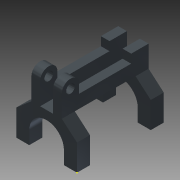
# Autodesk Inventor part: HW 4 Part 4
Saved by Autodesk Inventor 2015 (Build 190159000, 159)
## iProperties
Created: 2016-01-31
Part Number: HW 4 Part 4
Material: Iron, Cast
Document SubType Name: Modeling
Designer: Melissa
Mass: 1308.22 g
Surface Area: 443.91 cm^2
Volume: 182.968 cm^3
Density: 7.15 g/cm^3
Appearance: Iron Gray
Author: Melissa
Autodesk Inventor part; units mm, degrees
ref_plane "YZ Plane" through (0, 0, 0) normal (1, 0, 0) x (0, 1, 0)
ref_plane "XZ Plane" through (0, 0, 0) normal (0, 1, 0) x (-1, 0, 0)
ref_plane "XY Plane" through (0, 0, 0) normal (0, 0, 1) x (1, 0, 0)
sketch "Sketch1" plane through (0, 0, 0) normal (0, 0, 1) x (1, 0, 0)
  line L0 (0, 0) -> (19.05, 0)
  line L1 (19.05, 0) -> (19.05, 19.05)
  line L2 (69.85, 19.05) -> (69.85, 0)
  line L3 (69.85, 0) -> (88.9, 0)
  line L4 (88.9, 0) -> (88.9, 38.1)
  line L5 (88.9, 38.1) -> (66.675, 57.15)
  line L6 (66.675, 57.15) -> (22.225, 57.15)
  line L7 (22.225, 57.15) -> (0, 38.1)
  line L8 (0, 38.1) -> (0, 0)
  arc A0 (69.85, 19.05) -> (19.05, 19.05) centre (44.45, 19.05) ccw
  dimension "d0" = 38.1
  dimension "d1" = 44.45
  dimension "d2" = 88.9
  dimension "d3" = 19.05
  dimension "d5" = 19.05
  dimension "d6" = 19.05
  constraints: 18 end point, 3 equal length, 2 parallel, 2 perpendicular, 2 point on circle, 2 point on line, 1 centre point, 1 horizontal
  measures "d0" distance of L7.end L0.start
  measures "d1" distance of L5.end L6.end
  measures "d2" distance of L3.end L0.start
  measures "d3" distance of L0.start L0.end
  measures "d5" distance of L0.end L1.end
  measures "d6" vertical distance of L7.end L6.end
extrude "Extrusion1" add sketch "Sketch1" against normal blind 127
sketch "Sketch2" plane through (22.225, 57.15, 0) normal (0, 1, 0) x (1, 0, 0)
  line L0 (-22.225, 19.05) -> (68.7148, 19.05)
  line L1 (-22.225, 0) -> (-22.225, 127) projected
  line L2 (-22.225, 107.95) -> (68.7148, 107.95)
  line L3 (68.7148, 107.95) -> (68.7148, 19.05)
  line L4 (-22.225, 19.05) -> (-22.225, 107.95)
  line L5 (44.45, 0) -> (0, 0) projected
  line L6 (0, 127) -> (44.45, 127) projected
  dimension "d9" = 19.05
  dimension "d10" = 19.05
  constraints: 8 end point, 2 perpendicular, 1 collinear, 1 horizontal, 1 point on line
  measures "d9" distance between parallel lines of L0 L5
  measures "d10" distance between parallel lines of L6 L2
extrude "Extrusion2" cut sketch "Sketch2" against normal through all
sketch "Sketch3" plane through (88.9, 0, 0) normal (1, 0, 0) x (0, 0, -1)
  point P0 (0, 0)
sketch "Sketch4" plane through (88.9, 0, 0) normal (1, 0, 0) x (0, 0, -1)
  line L0 (0, 57.15) -> (0, 88.9)
  line L1 (25.4, 88.9) -> (25.4, 76.2)
  line L2 (25.4, 76.2) -> (101.6, 76.2)
  line L3 (101.6, 76.2) -> (101.6, 88.9)
  line L4 (101.6, 88.9) -> (127, 88.9)
  line L5 (127, 88.9) -> (127, 57.15)
  line L6 (127, 57.15) -> (0, 57.15)
  arc A0 (25.4, 88.9) -> (0, 88.9) centre (12.7, 88.9) ccw
  circle A1 centre (12.7, 88.9) radius 6.35
  point P0 (0, 0)
  dimension "d13" = 31.75
  dimension "d14" = 25.4
  dimension "d15" = 12.7
  dimension "d17" = 12.7
  constraints: 14 end point, 4 perpendicular, 2 centre point, 2 point on circle, 2 vertical, 1 parallel
  measures "d13" distance of L0.start L0.end
  measures "d14" distance of L3.end L4.end
  measures "d15" distance of L1.start L1.end
  measures "d17" diameter of A1
extrude "Extrusion3" add sketch "Sketch4" against normal blind 88.9
sketch "Sketch5" plane through (0, 0, 0) normal (0, 0, 1) x (1, 0, 0)
  line L0 (22.225, 104.8309) -> (22.225, 46.8186)
  line L1 (66.675, 46.8186) -> (66.6601, 105.2632)
  line L2 (0, 57.15) -> (0, 88.9) projected
  line L3 (22.225, 104.8309) -> (0, 104.8309)
  line L4 (0, 104.8309) -> (0, 57.15)
  line L5 (22.225, 57.15) -> (22.225, 104.8309)
  line L6 (66.6601, 105.2632) -> (88.8851, 105.2632)
  line L7 (88.8851, 105.2632) -> (88.8851, 57.15)
  line L8 (88.8851, 57.15) -> (66.675, 57.15)
  line L9 (0, 57.15) -> (22.225, 57.15)
  line L10 (22.225, 57.15) -> (0, 57.15) projected
  line L11 (88.9, 57.15) -> (66.675, 57.15) projected
  line L12 (66.6601, 105.2632) -> (88.9, 105.2632)
  line L13 (88.9, 105.2632) -> (88.9, 57.15)
  line L14 (88.9, 57.15) -> (66.6601, 57.15)
  line L15 (66.6601, 57.15) -> (66.6601, 105.2632)
  point P0 (0, 0)
  dimension "d20" = 22.225
  dimension "d21" = 44.45
  constraints: 26 end point, 4 horizontal, 4 parallel, 2 perpendicular, 1 collinear, 1 point on line, 1 vertical
  measures "d20" distance between parallel lines of L2 L0
  measures "d21" distance of L0.end L1.start
extrude "Extrusion4" cut sketch "Sketch5" against normal through all
sketch "Sketch6" plane through (0, 0, 0) normal (0, 0, 1) x (1, 0, 0)
  line L0 (66.6601, 57.15) -> (22.225, 57.15) projected
  line L1 (34.925, 57.15) -> (34.925, 106.1689)
  line L2 (34.925, 106.1689) -> (53.975, 106.1689)
  line L3 (53.975, 106.1689) -> (53.975, 57.15)
  line L4 (22.225, 88.9) -> (22.225, 57.15) projected
  point P0 (0, 0)
  dimension "d24" = 19.05
  dimension "d25" = 12.7
  constraints: 6 end point, 2 perpendicular, 2 point on line, 1 vertical
  measures "d24" distance between parallel lines of L3 L1
  measures "d25" distance between parallel lines of L1 L4
extrude "Extrusion5" cut sketch "Sketch6" against normal through all
body "Solid1"
